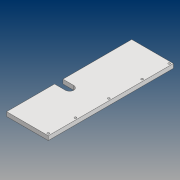
# Autodesk Inventor part: 08_Tam_canh_hong
Saved by Autodesk Inventor 2021 (Build 250183000, 183)
## iProperties
Created: 2024-04-01
Part Number: 08_Tam_canh_hong
Material: Generic
Document SubType Name: Modeling
Designer: Admin
Density: 1 g/cm^3
Appearance: Default
Author: Admin
Autodesk Inventor part; units mm, degrees
ref_plane "YZ Plane" through (0, 0, 0) normal (1, 0, 0) x (0, 1, 0)
ref_plane "XZ Plane" through (0, 0, 0) normal (0, 1, 0) x (-1, 0, 0)
ref_plane "XY Plane" through (0, 0, 0) normal (0, 0, 1) x (1, 0, 0)
sketch "Sketch1" plane through (0, 0, 0) normal (0, 1, 0) x (-1, 0, 0)
  line L0 (-50, 150) -> (50, 150)
  line L1 (50, 150) -> (50, -150)
  line L2 (50, -150) -> (-50, -150)
  line L3 (-50, -150) -> (-50, 150)
  line L4 (-50, 150) -> (50, -150) construction
  line L5 (50, 150) -> (-50, -150) construction
  point P0 (0, 0)
  dimension "d0" = 300
  dimension "d1" = 100
  constraints: 12 end point, 2 midpoint, 2 parallel, 1 horizontal, 1 perpendicular
  measures "d0" distance of L0.end L1.end
  measures "d1" distance between parallel lines of L1 L3
extrude "Extrusion1" add sketch "Sketch1" along normal blind 10
sketch "Sketch2" plane through (0, 0, 0) normal (0, -1, 0) x (1, 0, 0)
  circle A0 centre (-24, 25) radius 5 projected
  circle A1 centre (-24, 25) radius 10
  line L0 (-24, 35) -> (-24, 15)
  line L1 (-24, 15) -> (-50, 15)
  line L2 (-50, 15) -> (-50, 35)
  line L3 (-50, 35) -> (-24, 35)
  line L4 (-50, 200) -> (-50, -150) projected
  point P0 (0, 0)
  dimension "d4" = 20
  constraints: 8 end point, 2 parallel, 2 point on circle, 1 centre point, 1 coincident, 1 perpendicular, 1 point on line, 1 tangent, 1 vertical
  measures "d4" diameter of A1
extrude "Extrusion2" cut sketch "Sketch2" against normal blind 10
sketch "Sketch3" plane through (0, 0, 0) normal (0, -1, 0) x (1, 0, 0)
  line L0 (50, 150) -> (50, -150) projected
  line L1 (45, 150) -> (45, -150)
  line L2 (0, 0) -> (31.7101, 0) construction
  line L3 (-50, 150) -> (50, 150) projected
  point P0 (45, 0)
  point P1 (45, 145)
  point P2 (45, 80)
  point P3 (45, -80)
  point P4 (45, -145)
  dimension "d7" = 5
  dimension "d8" = 5
  dimension "d9" = 80
  constraints: 4 end point, 4 point on line, 2 symmetric about line, 1 horizontal, 1 midpoint, 1 parallel
  measures "d7" distance between parallel lines of L0 L1
  measures "d8" distance from line of L3 point (45, 145)
  measures "d9" distance of point (45, 0) point (45, 80)
hole "Hole1" at (45, 0, 0) at (45, 0, 145) at (45, 0, 80) at (45, 0, -80) at (45, 0, -145) direction (0, 1, 0) diameter 5 end through all
body "Solid1"
